Orbital Shaker movingPlatform_v22 (Autodesk Fusion 360 design; units mm, degrees)
Autodesk Fusion 360 part; units mm, degrees
sketch "movingPlatform" plane through (0, 0, 0) normal (0, 0, 1) x (1, 0, 0)
  line L0 (-75, 59) -> (75, 59)
  line L1 (75, 59) -> (75, -59)
  line L2 (75, -59) -> (-75, -59)
  line L3 (-75, -59) -> (-75, 59)
  line L4 (-75, 59) -> (75, -59) construction
  line L5 (75, 59) -> (-75, -59) construction
  circle A0 centre (-60, -34) radius 6.4
  line L6 (0, 2.5) -> (0, 20)
  circle A1 centre (60, -34) radius 6.4
  circle A2 centre (0, 34) radius 6.4
  circle A3 centre (-46, -46) radius 1.588
  circle A4 centre (-15.5, -15.5) radius 1.588
  circle A5 centre (0, 0) radius 57 construction
  circle A6 centre (15.5, -15.5) radius 1.588
  circle A7 centre (15.5, 15.5) radius 1.588
  circle A8 centre (46, -46) radius 1.588
  circle A9 centre (-46, 46) radius 1.588
  circle A10 centre (46, 46) radius 1.588
  circle A11 centre (-15.5, 15.5) radius 1.588
  dimension "d1" = 150
  dimension "d2" = 118
  dimension "d3" = 12.8
  dimension "d4" = 120
  dimension "d5" = 12.8
  dimension "d6" = 68
  dimension "d7" = 25
  dimension "d8" = 25
  dimension "d9" = 3.176
  dimension "d12" = 92
  dimension "d13" = 92
  dimension "d21" = 3.176
  dimension "d24" = 31
  dimension "d25" = 31
  dimension "d27" = 15.5
  dimension "d31" = 114
  dimension "d34" = 46
  dimension "d37" = 46
  dimension "d49" = 15.5
  constraint horizontal L0
  constraint perpendicular L0 L1
  constraint parallel L0 L2
  constraint parallel L1 L3
  constraint coincident L4 A5.centre
  constraint coincident L5 A5.centre
  constraint coincident A5.centre origin
  constraint symmetric A0 L6 A1
  constraint coincident L6 A2.centre
  measures "d1" distance of L0.start L0.end
  measures "d2" distance of L0.start L2.end
  measures "d3" diameter of A0
  measures "d4" distance of A0.centre A1.centre
  measures "d5" diameter of A2
  measures "d6" vertical distance of A0.centre A2.centre
  measures "d7" distance of L2 A1.centre
  measures "d8" distance of L0 A2.centre
  measures "d9" diameter of A3
  measures "d21" diameter of A4
  measures "d27" horizontal distance of A5.centre A4.centre
  measures "d31" diameter of A5
  measures "d34" vertical distance of A3.centre A5.centre
  measures "d37" horizontal distance of A3.centre A5.centre
  measures "d49" vertical distance of A5.centre A4.centre
extrude "Extrude3" add sketch "movingPlatform" along normal blind 3.175
equation "d4 = 132.800 mm - 12.8 mm"
